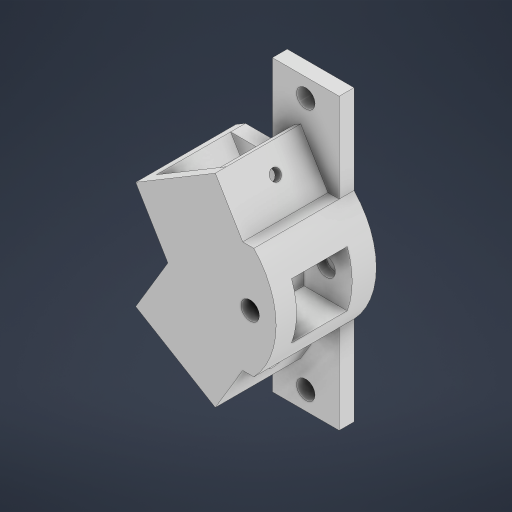
# Autodesk Inventor part: 2020_top_guide_mnt
Saved by Autodesk Inventor 2024 (Build 280153000, 153)
## iProperties
Created: 2026-03-27
Part Number: 2020_top_guide_mnt
Material: PET Plastic
Document SubType Name: Modeling
Designer: schar
Density: 1.541 g/cm^3
Appearance: Polycarbonate - Clear
Mass: 30.1405 g
Surface Area: 121.903 cm^2
Volume: 19.559 cm^3
Author: schar
Autodesk Inventor part; units mm, degrees
ref_plane "YZ Plane" through (0, 0, 0) normal (1, 0, 0) x (0, 1, 0)
sketch "Sketch1" plane through (0, 0, 0) normal (0, 0, 1) x (1, 0, 0)
  circle A0 centre (-0.0001, 55.0001) radius 2.5 projected
  line L0 (-9, 60.0001) -> (-9, 34.0001) projected
  line L1 (-9, 34.0001) -> (-5.0001, 34.0001) projected
  line L2 (-5.0001, 34.0001) -> (-5.0001, 45.0001) projected
  line L3 (-5.0001, 45.0001) -> (4.9999, 45.0001) projected
  line L4 (4.9999, 45.0001) -> (4.9999, 34.0001) projected
  line L5 (4.9999, 34.0001) -> (8.9999, 34.0001) projected
  line L6 (8.9999, 34.0001) -> (8.9999, 60.0001) projected
  line L7 (8.9999, 60.0001) -> (-9, 60.0001) projected
  line L8 (-9, 8) -> (-9, -18) projected
  line L9 (-5, -18) -> (-5, -8) projected
  circle A1 centre (-0.0001, -13.0001) radius 2.5 projected
  line L10 (8.9999, -18.0001) -> (8.9999, 7.9999) projected
  line L11 (8.9999, 7.9999) -> (4.9999, 7.9999) projected
  line L12 (4.9999, 7.9999) -> (4.9999, 2.5001) projected
  line L13 (5, -3) -> (-5.0001, -3.0001) projected
  line L14 (-5.0001, -3.0001) -> (-5.0001, 7.9999) projected
  line L15 (-5.0001, 7.9999) -> (-9, 7.9999) projected
  line L16 (-9, -18.0001) -> (8.9999, -18.0001) projected
  line L17 (8.9999, 60.0001) -> (-9, 60.0001)
  line L18 (-9, 60.0001) -> (-9, -18)
  line L19 (-9, -18) -> (8.9999, -18)
  line L20 (8.9999, -18) -> (8.9999, 60.0001)
  circle A2 centre (-0.0001, 55.0001) radius 2.5
  circle A3 centre (-0.0001, -13.0001) radius 2.5
  line L21 (-9, 7.9999) -> (-9, -18.0001) projected
  line L22 (4.9999, 2.5001) -> (5, -3) projected
  point P0 (0, 0)
  dimension "d0" = 4
  dimension "d1" = 0
  constraints: 8 end point, 2 centre point, 2 coincident, 2 concentric, 2 parallel, 1 horizontal, 1 perpendicular, 1 other
extrude "Extrusion1" add sketch "Sketch1" along normal blind 4
sketch "Sketch2" plane through (0, 0, 4) normal (0, 0, 1) x (1, 0, 0)
  circle A0 centre (-55.3, -73.0192) radius 2.5 projected
  circle A1 centre (-55.3001, 115.0193) radius 2.5 projected
  line L0 (-55.3, -73.0192) -> (33.584, 75.4143)
  line L1 (-55.3001, 115.0193) -> (26.1085, -20.9304)
  line L2 (-9, 60) -> (-9, -18) projected
  line L3 (-9, 21) -> (62.9573, 21)
  line L4 (1, 21) -> (-7.5794, 15.8625)
  line L5 (-55.3001, 115.0193) -> (-50.1626, 106.4399)
  line L6 (-50.1626, 106.4399) -> (-41.5832, 111.5774)
  line L7 (-50.1626, 106.4399) -> (-58.742, 101.3024)
  line L8 (-7.5794, 15.8625) -> (-58.742, 101.3024)
  line L9 (1, 21) -> (9.5794, 26.1375)
  line L10 (9.5794, 26.1375) -> (-41.5832, 111.5774)
  line L11 (1, 21) -> (-7.5794, 26.1375)
  line L12 (1, 21) -> (9.5794, 15.8625)
  line L13 (-55.3, -73.0192) -> (-50.1625, -64.4398)
  line L14 (-93.1275, -68.5) -> (-47.8, -94.6699) projected
  line L15 (-50.1625, -64.4398) -> (-41.5831, -69.5773)
  line L16 (-50.1625, -64.4398) -> (-58.742, -59.3023)
  line L17 (-41.5831, -69.5773) -> (9.5794, 15.8625)
  line L18 (-7.5794, 26.1375) -> (-58.742, -59.3023)
  line L19 (-10.6558, 21) -> (6.503, 31.2749)
  line L20 (-10.6558, 21) -> (6.503, 10.7251)
  circle A2 centre (-0.0001, -13.0001) radius 2.5 projected
  circle A3 centre (-0.0001, -13.0001) radius 5
  circle A4 centre (-0.0001, 55.0001) radius 2.5 projected
  circle A5 centre (-0.0001, 55.0001) radius 5
  line L21 (8.9999, 60.0001) -> (-9, 60.0001) projected
  line L22 (-9, -18.0001) -> (8.9999, -18.0001) projected
  line L23 (-20.2607, 4.9602) -> (12.7451, -14.8042)
  line L24 (-20.2607, 37.0398) -> (12.7451, 56.8042)
  line L25 (-20.2607, 4.9602) -> (-22.8345, 6.5014)
  line L26 (-9, 21) -> (-33.1607, 21)
  line L27 (-22.8345, 6.5014) -> (-14.1525, 21)
  line L28 (-20.2607, 37.0398) -> (-22.8345, 35.4986)
  line L29 (-22.8345, 35.4986) -> (-14.1525, 21)
  line L30 (6.503, 10.7251) -> (8.9999, 9.2299)
  line L31 (8.9999, -18.0001) -> (8.9999, 60.0001) projected
  line L32 (6.503, 31.2749) -> (8.9999, 32.7701)
  line L33 (8.9999, 32.7701) -> (-0.605, 48.8099)
  line L34 (8.9999, 9.2299) -> (-0.605, -6.8099)
  line L35 (8.9999, 32.7701) -> (8.9999, 9.2299)
  line L36 (-22.8345, 6.5014) -> (-22.8345, 35.4986)
  point P0 (0, 0)
  point P1 (-20.2607, 37.0398)
  point P2 (6.503, 10.7251)
  point P3 (-3.1018, -5.3148)
  point P4 (8.524, 8.4352)
  point P5 (7.516, 10.1185)
  point P6 (-3.1019, 47.3148)
  point P7 (6.503, 31.2749)
  point P8 (-2.0764, 26.1375)
  point P9 (-11.6813, 42.1773)
  point P10 (6.8279, 11.2676)
  point P11 (8.9999, 14.8947)
  point P12 (8.9999, 16.2096)
  point P13 (6.503, 10.7251)
  point P14 (8.9999, 25.7904)
  point P15 (6.503, 31.2749)
  point P16 (8.9999, 27.1053)
  point P17 (8.9999, 32.7701)
  point P18 (8.9999, 32.7704)
  point P19 (8.9999, 9.2299)
  point P20 (8.9999, 7.6404)
  point P21 (8.9999, 9.2296)
  point P22 (8.9999, 54.5615)
  point P23 (8.9999, -12.5615)
  dimension "d0" = 4
  dimension "d1" = 0
  dimension "d2" = 10
  dimension "d3" = 10
  dimension "d4" = 10
  dimension "d5" = 10
  dimension "d6" = 10
  dimension "d7" = 10
  dimension "d8" = 10
  dimension "d9" = 10
  dimension "d10" = 10
  dimension "d11" = 10
  dimension "d12" = 10
  dimension "d13" = 20
  dimension "d14" = 20
  dimension "d15" = 3
  dimension "d16" = 3
  constraints: 64 end point, 13 point on line, 12 perpendicular, 4 parallel, 3 collinear, 2 centre point, 2 coincident, 2 horizontal, 2 midpoint, 2 symmetric about line, 1 tangent, 4 other
  measures "d2" distance of L26.start L4.start
  measures "d3" distance of L4.start L4.end
  measures "d4" distance of L1.start L5.end
  measures "d5" distance of L5.end L6.end
  measures "d6" distance of L5.end L7.end
  measures "d7" distance of L4.start L9.end
  measures "d8" distance of L4.start L11.end
  measures "d9" distance of L4.start L12.end
  measures "d10" distance of L0.start L13.end
  measures "d11" distance of L13.end L15.end
  measures "d12" distance of L13.end L16.end
  measures "d13" distance of L19.start L19.end
  measures "d14" distance of L19.start L20.end
  measures "d15" distance of L23.start L25.end
  measures "d16" distance of L24.start L28.end
extrude "Extrusion2" add sketch "Sketch2" along normal blind 20 contours L25 L27 L26 L18 | L20 L4 L0 | L0 L1 L17 L20 | L26 L29 L28 L8 | L26 L2 L20 | L19 L2 L26 | L17 L30 L1 L34 L23 | L1 L19 L10 L0 | L11 L19 L1 | L12 L31 L17 L1 | L4 L20 L2 L3 | L9 L31 L3 | L0 L10 L31 L9 | L3 L2 L19 L11 | L3 L31 L12 | L17 L1 L30 | L34 L1 L31 L23 | L10 L32 L0 | L0 L32 L31 L10 | L17 L31 L30 L1 | L30 L34 L1 | L34 L31 L1 | L32 L10 L24 L33 L0 | L0 L33 L32 | L33 L24 L31 L0 | L0 L31 L33
sketch "Sketch3" plane through (0, 0, 4) normal (0, 0, -1) x (-1, 0, 0)
  line L0 (10.6558, 21) -> (20.2607, 37.0398) projected
  line L1 (20.2607, 37.0398) -> (8.9915, 37.0398)
  line L2 (20.2607, 4.9602) -> (10.6558, 21) projected
  line L3 (20.2607, 4.9602) -> (9, 4.9602)
  line L4 (9, 20.0085) -> (9, -18) projected
  line L5 (22.8345, 35.4986) -> (14.1525, 21) projected
  line L6 (22.8345, 6.5014) -> (20.2607, 4.9602) projected
  line L7 (22.8345, 35.4986) -> (22.8345, 6.5014)
  line L8 (9, 60) -> (9, -18) projected
  line L9 (10.6558, 21) -> (9, 20.0085) projected
  line L10 (9, 21.9915) -> (10.6558, 21) projected
  line L11 (22.8345, 6.5014) -> (20.2607, 4.9602) projected
  line L12 (14.1525, 21) -> (22.8345, 6.5014) projected
  line L13 (22.8345, 35.4986) -> (14.1525, 21) projected
  line L14 (20.2607, 37.0398) -> (22.8345, 35.4986) projected
  line L15 (10.6558, 21) -> (20.2607, 37.0398) projected
  line L16 (20.2607, 4.9602) -> (10.6558, 21) projected
  line L17 (-8.9999, 60.0001) -> (9, 60.0001) projected
  line L18 (-8.9999, -18.0001) -> (-8.9999, 60.0001) projected
  line L19 (9, -18.0001) -> (-8.9999, -18.0001) projected
  circle A0 centre (0.0001, -13.0001) radius 2.5 projected
  circle A1 centre (0.0001, 55.0001) radius 2.5 projected
  line L20 (9, 60.0001) -> (9, -18.0001) projected
  point P0 (0, 0)
  point P1 (9, 37.0398)
  dimension "d0" = 4
  dimension "d1" = 0
  constraints: 6 end point, 2 horizontal, 1 point on line, 1 vertical
ref_plane "Work Plane1" through (-20.2583, -25.7942, 0) normal (0, 0, 1) x (1, 0, 0)
extrude "Extrusion3" add sketch "Sketch3" along normal up to surface (4 mm away) contours L10 L8 L1 L0 | L0 L14 L5 L12 L6 L2 | L2 L3 L4 L9 | L9 L8 L10 | L7 L12 L5
ref_plane "Work Plane4" through (8.9999, -18.0001, 0) normal (1, 0, 0) x (0, 0, -1)
sketch "Sketch12" plane through (0, 0, 24) normal (0, 0, 1) x (1, 0, 0)
  line L0 (-3.1018, -5.3148) -> (8.9999, -12.5615) projected
  line L1 (-14.1525, 21) -> (-22.8345, 6.5014) projected
  line L2 (8.9999, -12.5615) -> (-22.8345, 6.5014)
  line L3 (-22.8345, 6.5014) -> (-14.1525, 21)
  line L4 (-22.8345, 35.4986) -> (-14.1525, 21) projected
  line L5 (-14.1525, 21) -> (-22.8345, 35.4986)
  line L6 (-22.8345, 35.4986) -> (8.9999, 54.5615)
  line L7 (8.9999, 54.5615) -> (8.9999, -12.5615)
  point P0 (0, 0)
  constraints: 10 end point, 2 collinear, 2 perpendicular, 1 vertical
extrude "Extrusion12" add sketch "Sketch12" along normal blind 3
sketch "Sketch13" plane through (0, 0, 27) normal (0, 0, 1) x (1, 0, 0)
  line L0 (8.9999, -12.5615) -> (8.9999, 54.5615) projected
  line L1 (8.9999, 21) -> (14.9999, 21)
  line L2 (8.9999, 21) -> (8.9999, 6)
  line L3 (8.9999, 21) -> (8.9999, 36)
  arc A0 (8.9999, 6) -> (8.9999, 36) centre (-6.7501, 21) ccw
  point P0 (0, 0)
  dimension "d52" = 6
  dimension "d53" = 15
  dimension "d54" = 15
  constraints: 6 end point, 3 point on circle, 2 point on line, 1 centre point, 1 horizontal, 1 midpoint
  measures "d52" distance of L1.start L1.end
  measures "d53" distance of L1.start L2.end
  measures "d54" distance of L1.start L3.end
extrude "Extrusion13" add sketch "Sketch13" against normal up to surface (27 mm away)
sketch "Sketch14" plane through (0, 0, 27) normal (0, 0, 1) x (1, 0, 0)
  arc A0 (8.9999, 6) -> (8.9999, 36) centre (-6.7501, 21) ccw projected
  line L0 (14.9999, 21) -> (7.9999, 21)
  circle A1 centre (7.9999, 21) radius 2.5
  point P0 (0, 0)
  dimension "d57" = 7
  dimension "d58" = 5
  constraints: 2 end point, 1 centre point, 1 coincident, 1 horizontal, 1 point on circle
  measures "d57" distance of L0.start L0.end
  measures "d58" diameter of A1
extrude "Extrusion14" cut sketch "Sketch14" against normal up to surface (23 mm away)
sketch "Sketch15" plane through (8.9999, -18.0001, 4) normal (1, 0, 0) x (0, 0, -1)
  line L0 (-23, 54.0001) -> (-23, 24.0001) projected
  line L1 (-23, 39.0001) -> (-10, 39.0001)
  line L2 (0, 39.0001) -> (-20, 39.0001) projected
  line L3 (-17.5, 31.5001) -> (-2.5, 31.5001)
  line L4 (-2.5, 31.5001) -> (-2.5, 46.5001)
  line L5 (-2.5, 46.5001) -> (-17.5, 46.5001)
  line L6 (-17.5, 46.5001) -> (-17.5, 31.5001)
  line L7 (-17.5, 31.5001) -> (-2.5, 46.5001) construction
  line L8 (-2.5, 31.5001) -> (-17.5, 46.5001) construction
  point P0 (4, 18.0001)
  dimension "d61" = 15
  dimension "d62" = 15
  constraints: 14 end point, 4 midpoint, 2 parallel, 1 horizontal, 1 perpendicular
  measures "d61" distance of L5.end L4.end
  measures "d62" distance of L4.end L3.end
extrude "Extrusion15" cut sketch "Sketch15" along normal blind 10 and the other way blind 7
sketch "Sketch16" plane through (0, 0, 27) normal (0, 0, 1) x (1, 0, 0)
  line L0 (-3.1018, -5.3148) -> (6.503, 10.7251) projected
  line L1 (6.503, 31.2749) -> (-3.1019, 47.3148) projected
  line L2 (-3.1018, -5.3148) -> (-1.386, -6.3423)
  line L3 (-22.8345, 6.5014) -> (8.9999, -12.5615) projected
  line L4 (-1.386, -6.3423) -> (4.4507, 3.4048)
  line L5 (8.9999, -12.5615) -> (8.9999, 6) projected
  line L6 (8.9999, 6) -> (-9.8503, 6)
  line L7 (4.4507, 3.4048) -> (6.0048, 6)
  line L8 (-22.8345, 35.4986) -> (-14.1525, 21) projected
  line L9 (-14.1525, 21) -> (17.1457, 21)
  line L10 (-22.8345, 35.4986) -> (8.9999, 54.5615)
  line L11 (-1.386, 48.3423) -> (4.4507, 38.5952)
  line L12 (8.9999, 54.5615) -> (8.9999, 36)
  line L13 (8.9999, 36) -> (-9.8503, 36)
  line L14 (4.4507, 38.5952) -> (6.0048, 36)
  point P0 (0, 0)
  dimension "d67" = 2
  constraints: 20 end point, 6 symmetric about line, 3 point on line, 2 horizontal, 1 collinear, 1 perpendicular, 1 other
  measures "d67" distance of L0.start L2.end
extrude "Extrusion16" cut sketch "Sketch16" against normal up to surface (23 mm away) contours L4 L7 L6 L5 L3 | L14 L11 L10 L12 L13
sketch "Sketch17" plane through (6.0048, 6, 27) normal (0.8579416, -0.5137472, 0) x (0, 0, -1)
  line L0 (0, 2.5134) -> (0, -14.3859) projected
  line L1 (0, -8.2326) -> (13, -8.2326)
  circle A0 centre (13, -8.2326) radius 1.5
  point P0 (27, -8.2326)
  dimension "d71" = 13
  dimension "d72" = 3
  constraints: 2 end point, 1 centre point, 1 coincident, 1 perpendicular, 1 point on line
  measures "d71" distance of L1.start L1.end
  measures "d72" diameter of A0
extrude "Extrusion17" cut sketch "Sketch17" against normal through all
sketch "Sketch18" plane through (6.0048, 36, 27) normal (0.8579416, 0.5137472, 0) x (0, 0, -1)
  line L0 (23, 14.3859) -> (0, 14.3859) projected
  line L1 (0, 14.3859) -> (0, 8.2329)
  line L2 (0, 14.3859) -> (0, -2.5134) projected
  line L3 (0, 8.2329) -> (13, 8.2329)
  circle A0 centre (13, 8.2329) radius 1.5
  point P0 (27, -27.801)
  dimension "d75" = 6.153
  dimension "d76" = 13
  dimension "d77" = 3
  constraints: 4 end point, 1 centre point, 1 coincident, 1 perpendicular, 1 point on line
  measures "d75" distance of L0.end L1.end
  measures "d76" distance of L1.end L3.end
  measures "d77" diameter of A0
extrude "Extrusion18" cut sketch "Sketch18" against normal through all
body "Solid1"
